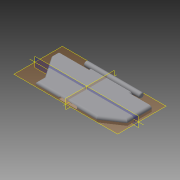
# Autodesk Inventor part: ChassisRechtsUntenKlappe
Saved by Autodesk Inventor 2015 (Build 190159000, 159)
## iProperties
Created: 2018-11-29
Part Number: ChassisRechtsUntenKlappe
Material: Generisch
Document SubType Name: Modeling
Designer: Boris
Density: 1 g/cm^3
Appearance: Vorgabe
Author: Boris
Autodesk Inventor part; units mm, degrees
sketch "Skizze1" plane through (0, 0, 0) normal (0, 0, 1) x (1, 0, 0)
  line L0 (-38.5, 9.6694) -> (-38.5, 14.6694)
  line L1 (-26.5, -7.8306) -> (-38.5, 9.6694)
  line L2 (-26.5, -15.3306) -> (-26.5, -7.8306)
  line L3 (23.5, -15.3306) -> (-26.5, -15.3306)
  line L4 (38.5, -5.3306) -> (23.5, -15.3306)
  line L5 (38.5, 14.6694) -> (38.5, -5.3306)
  line L6 (-38.5, 14.6694) -> (38.5, 14.6694)
  line L7 (0, 48.0661) -> (0, -25.8968) projected
  point P0 (0, 0)
  point P1 (40.5, 37.5)
  dimension "d0" = 77
  dimension "d1" = 20
  dimension "d2" = 50
  dimension "d3" = 5
  dimension "d4" = 15
  dimension "d5" = 17.5
  dimension "d6" = 7.5
  constraints: 14 end point, 2 parallel, 2 perpendicular, 1 symmetric about line
  measures "d0" distance of L0.end L5.start
  measures "d1" distance of L5.start L4.start
  measures "d2" distance of L3.start L2.start
  measures "d3" distance of L0.start L0.end
  measures "d4" horizontal distance of L4.start L3.start
  measures "d5" vertical distance of L1.start L0.start
  measures "d6" distance of L2.start L1.start
extrude "Extrusion1" add sketch "Skizze1" along normal mid plane 4
sketch "Skizze2" plane through (-26.5, -15.3306, 2) normal (0, -1, 0) x (1, 0, 0)
  line L0 (26.5, -4.8) -> (26.5, 0.8) projected
  line L1 (-27.4, -2) -> (80.4, -2) projected
  line L2 (34, -3) -> (19, -3)
  line L3 (19, -3) -> (19, -1)
  line L4 (19, -1) -> (34, -1)
  line L5 (34, -1) -> (34, -3)
  point P0 (26.5, -2)
  dimension "d9" = 15
  dimension "d10" = 2
  constraints: 8 end point, 2 parallel, 1 horizontal, 1 perpendicular, 2 other
  measures "d9" distance of L3.end L4.end
  measures "d10" distance of L2.end L3.end
extrude "Extrusion2" cut sketch "Skizze2" against normal blind 10
fillet "Rundung1" radius 1 4 edges at (7.5, -10.3306, 1) (7.5, -10.3306, -1) (-7.5, -10.3306, 1) (-7.5, -10.3306, -1)
sketch "Skizze3" plane through (0, 0, -2) normal (0, 0, -1) x (-1, 0, 0)
  line L0 (-6.5, -5.3306) -> (6.5, -5.3306) projected
  line L1 (-6.5, -5.3306) -> (-6.5, -15.3306) projected
  line L2 (6.5, -15.3306) -> (6.5, -5.3306) projected
  line L3 (7.5, -5.3306) -> (7.5, -15.3306) projected
  line L4 (6.5, -5.3306) -> (7.5, -5.3306) projected
  line L5 (-7.5, -5.3306) -> (-7.5, -15.3306) projected
  line L6 (-7.5, -5.3306) -> (-6.5, -5.3306) projected
  line L7 (0, -21.3306) -> (0, 20.6694) projected
  line L8 (-1.5, -6.3306) -> (1.5, -6.3306)
  line L9 (1.5, -6.3306) -> (1.5, -13.3306)
  line L10 (1.5, -13.3306) -> (-1.5, -13.3306)
  line L11 (-1.5, -13.3306) -> (-1.5, -6.3306)
  point P0 (0, 0)
  dimension "d14" = 3
  dimension "d15" = 7
  dimension "d74" = 1
  constraints: 8 end point, 2 parallel, 1 horizontal, 1 perpendicular, 1 other
  measures "d14" distance of L9.end L10.end
  measures "d15" distance of L8.end L9.end
  measures "d74" distance between parallel lines of L0 L8
extrude "Extrusion3" cut sketch "Skizze3" against normal blind 2
fillet "Rundung2" radius 0.5 4 edges at (1.5, -6.3306, -1.5) (-1.5, -6.3306, -1.5) (-1.5, -13.3306, -1.5) (1.5, -13.3306, -1.5)
sketch "Skizze4" plane through (0, 0, -2) normal (0, 0, -1) x (-1, 0, 0)
  line L0 (-31.5, 11.6694) -> (11.5, 11.6694)
  line L1 (11.5, 11.6694) -> (11.5, -5.3306)
  line L2 (11.5, -5.3306) -> (-31.5, -5.3306)
  line L3 (-31.5, -5.3306) -> (-31.5, 11.6694)
  line L4 (-23.5, -15.3306) -> (26.5, -15.3306) projected
  line L5 (-38.5, 14.6694) -> (38.5, 14.6694) projected
  line L6 (-38.5, 14.6694) -> (-38.5, -5.3306) projected
  line L7 (38.5, 9.6694) -> (38.5, 14.6694) projected
  point P0 (0, 0)
  dimension "d19" = 10
  dimension "d20" = 3
  dimension "d21" = 7
  dimension "d22" = 27
  constraints: 8 end point, 2 parallel, 1 horizontal, 1 perpendicular
  measures "d19" distance between parallel lines of L4 L2
  measures "d20" distance between parallel lines of L5 L0
  measures "d21" distance between parallel lines of L6 L3
  measures "d22" distance between parallel lines of L1 L7
extrude "Extrusion4" cut sketch "Skizze4" against normal blind 1
sketch "Skizze5" plane through (0, 0, -1) normal (0, 0, -1) x (-1, 0, 0)
  line L0 (-6.5, -5.3306) -> (-31.5, -5.3306) projected
  line L1 (-31.5, 11.6694) -> (-30.5, 11.6694)
  line L2 (-30.5, 11.6694) -> (-30.5, -5.3306)
  line L3 (-30.5, -5.3306) -> (-31.5, -5.3306)
  line L4 (-31.5, -5.3306) -> (-31.5, 11.6694)
  point P0 (0, 0)
  dimension "d25" = 1
  constraints: 8 end point, 2 parallel, 1 horizontal, 1 perpendicular, 1 point on line
  measures "d25" distance of L2.end L3.end
extrude "Extrusion5" add sketch "Skizze5" along normal blind 1
chamfer "Fase1" distance 1 angle 45 1 edges at (30.5, 3.1694, -2)
pattern_linear "Rechteckige Anordnung1" count 21 spacing 2.05 along (-1, 0, 0) of "Extrusion5", "Fase1"
sketch "Skizze6" plane through (0, 0, -2) normal (0, 0, -1) x (-1, 0, 0)
  circle A0 centre (-33.5, 10.4576) radius 0.75
  circle A1 centre (-33.5, -4.329) radius 0.75
  circle A2 centre (12.5, -4.329) radius 0.75
  circle A3 centre (12.5, 10.4576) radius 0.75
  line L0 (-31.5, 11.6694) -> (-31.5, -5.3306) projected
  line L1 (10.5, 11.6694) -> (10.5, -5.3306) projected
  point P0 (0, 0)
  dimension "d34" = 1.5
  dimension "d35" = 1.5
  dimension "d36" = 1.5
  dimension "d37" = 1.5
  dimension "d38" = 2
  dimension "d40" = 2
  dimension "d41" = 2
  dimension "d42" = 2
  constraints: 4 centre point
  measures "d34" diameter of A0
  measures "d35" diameter of A1
  measures "d36" diameter of A2
  measures "d37" diameter of A3
  measures "d38" distance from line of A0.centre L0
  measures "d40" distance from line of L0 A1.centre
  measures "d41" distance from line of L1 A3.centre
  measures "d42" distance from line of L1 A2.centre
extrude "Extrusion6" add sketch "Skizze6" along normal blind 1.5
fillet "Rundung3" radius 0.5 8 edges at (34.25, -4.329, -3.5) (34.25, 10.4576, -3.5) (-11.75, 10.4576, -3.5) (-11.75, -4.329, -3.5) (-11.75, -4.329, -2) (-11.75, 10.4576, -2) (34.25, -4.329, -2) (34.25, 10.4576, -2)
sketch "Skizze7" plane through (0, 0, -2) normal (0, 0, -1) x (-1, 0, 0)
  line L0 (-38.5, 14.6694) -> (38.5, 14.6694) projected
  line L1 (18.5, 14.6694) -> (18.5, -15.3306)
  line L2 (-23.5, -15.3306) -> (26.5, -15.3306) projected
  line L3 (26.5, -15.3306) -> (26.5, -7.8306) projected
  line L4 (19.5, 14.6694) -> (19.5, -15.3306)
  line L5 (18.5, 14.6694) -> (19.5, 14.6694)
  line L6 (19.5, -15.3306) -> (18.5, -15.3306)
  point P0 (0, 0)
  dimension "d46" = 8
  dimension "d47" = 1
  constraints: 8 end point, 2 parallel, 2 point on line, 1 horizontal, 1 vertical
  measures "d46" distance between parallel lines of L1 L3
  measures "d47" distance between parallel lines of L1 L4
extrude "Extrusion7" cut sketch "Skizze7" against normal blind 1
fillet "Rundung4" radius 0.5 4 edges at (-18.5, -0.3306, -1) (-19.5, -0.3306, -1) (-19.5, -0.3306, -2) (-18.5, -0.3306, -2)
fillet "Rundung6" radius 2 6 edges at (-38.5, 12.1694, 2) (-32.5, 0.9194, 2) (-1.5, -15.3306, 2) (-26.5, -11.5806, 2) (31, -10.3306, 2) (38.5, 4.6694, 2)
sketch "Skizze8" plane through (-18, 14.6694, -2) normal (0, 1, 0) x (1, 0, 0)
  line L0 (39, -4) -> (4, -4)
  line L1 (4, -4) -> (4, 0)
  line L2 (4, 0) -> (39, 0)
  line L3 (39, 0) -> (39, -4)
  line L4 (54.5, -4) -> (-18.5, -4) projected
  line L5 (56.5, -2) -> (56.5, 0) projected
  point P0 (18, -2)
  dimension "d53" = 35
  dimension "d54" = 4
  dimension "d55" = 0
  dimension "d56" = 17.5
  constraints: 8 end point, 2 parallel, 1 horizontal, 1 perpendicular
  measures "d53" distance of L1.end L2.end
  measures "d54" distance of L0.end L1.end
  measures "d55" distance between parallel lines of L4 L0
  measures "d56" distance between parallel lines of L5 L3
extrude "Extrusion8" add sketch "Skizze8" along normal blind 6
sketch "Skizze9" plane through (-14, 14.6694, -2) normal (-1, 0, 0) x (0, 0, 1)
  circle A0 centre (3.75, 3.5) radius 2
  line L0 (0, 0) -> (0, 6) projected
  line L1 (0, 6) -> (4, 6) projected
  point P0 (2, -14.6694)
  dimension "d59" = 4
  dimension "d60" = 3.75
  dimension "d61" = 2.5
  constraints: 1 centre point
  measures "d59" diameter of A0
  measures "d60" distance from line of L0 A0.centre
  measures "d61" distance from line of L1 A0.centre
extrude "Extrusion9" add sketch "Skizze9" along normal blind 5 and the other way blind 41
fillet "Rundung7" radius 2 1 edges at (3.5, 20.6694, 2)
fillet "Rundung8" radius 2 1 edges at (3.5, 20.6694, -2)
fillet "Rundung9" radius 2 1 edges at (3.5, 20.1537, 2)
fillet "Rundung13" radius 2 2 edges at (21, 15.4272, 2) (-14, 15.4272, 2)
fillet "Rundung14" radius 1 2 edges at (27, 18.1694, -0.25) (-19, 18.1694, -0.25)
